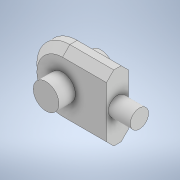
# Autodesk Inventor part: 2번부품
Saved by Autodesk Inventor 2022 (Build 260153000, 153)
## iProperties
Created: 2021-09-05
Part Number: 2번부품
Material: 일반
Document SubType Name: Modeling
Designer: 서울공업고등학교
Density: 1 g/cm^3
Appearance: 기본값
Author: 서울공업고등학교
Autodesk Inventor part; units mm, degrees
ref_plane "YZ Plane" through (0, 0, 0) normal (1, 0, 0) x (0, 1, 0)
ref_plane "XZ Plane" through (0, 0, 0) normal (0, 1, 0) x (-1, 0, 0)
ref_plane "XY Plane" through (0, 0, 0) normal (0, 0, 1) x (1, 0, 0)
sketch "스케치1" plane through (0, 0, 0) normal (0, 0, 1) x (1, 0, 0)
  circle A0 centre (0, 0) radius 3.5
  line L0 (-9, 9) -> (12, 9)
  line L1 (12, 9) -> (12, -9)
  line L2 (12, -9) -> (-9, -9)
  line L3 (-9, -9) -> (-9, 9)
  dimension "d0" = 7
  dimension "d1" = 21
  dimension "d2" = 18
  dimension "d3" = 12
  dimension "d4" = 9
  constraints: 8 end point, 2 parallel, 1 centre point, 1 coincident, 1 horizontal, 1 perpendicular
  measures "d0" diameter of A0
  measures "d1" distance of L0.start L0.end
  measures "d2" distance of L2.end L0.start
  measures "d3" distance from line of L1 point (0, 0)
  measures "d4" distance from line of point (0, 0) L0
extrude "돌출1" add sketch "스케치1" along normal mid plane 6
extrude "돌출2" add sketch "스케치1" along normal mid plane 15 contours A0
fillet "모깎기1" radius 9 2 edges at (-9, 9, 0) (-9, -9, 0)
chamfer "모따기1" distance 2 angle 45 6 edges at (-6.3641, 6.3641, 3) (5.9998, 9, 3) (5.9998, -9, 3) (-6.3641, 6.3641, -3) (5.9998, -9, -3) (5.9998, 9, -3)
sketch "스케치2" plane through (12, -7, 3) normal (1, 0, 0) x (0, 0, -1)
  circle A0 centre (3, 7) radius 2.5
  dimension "d13" = 5
  constraints: 1 centre point, 1 coincident
  measures "d13" diameter of A0
extrude "돌출3" add sketch "스케치2" along normal blind 6
